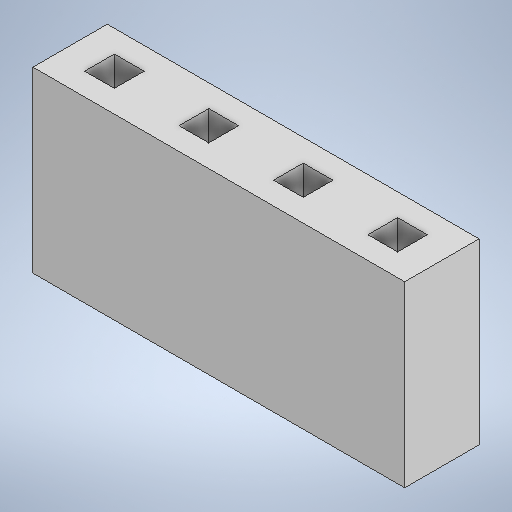
# Autodesk Inventor part: ikafly8_2.54
Saved by Autodesk Inventor 2025 (Build 290162000, 162)
## iProperties
Created: 2024-05-24
Part Number: ikafly8_2.54
Material: 一般
Document SubType Name: Modeling
Designer: Saigusa
Density: 1 g/cm^3
Appearance: 既定
Author: Saigusa
Autodesk Inventor part; units mm, degrees
ref_plane "YZ Plane" through (0, 0, 0) normal (1, 0, 0) x (0, 1, 0)
ref_plane "XZ Plane" through (0, 0, 0) normal (0, 1, 0) x (-1, 0, 0)
ref_plane "XY Plane" through (0, 0, 0) normal (0, 0, 1) x (1, 0, 0)
sketch "スケッチ1" plane through (0, 0, 0) normal (0, 1, 0) x (-1, 0, 0)
  line L0 (0, 0) -> (5.08, 0)
  line L1 (5.08, 0) -> (2.54, 0)
  line L2 (2.54, 0) -> (0, 0)
  line L3 (0, 0) -> (-2.54, 0)
  line L4 (-2.54, 0) -> (-5.08, 0)
  circle A0 centre (-2.54, 0) radius 0.4
  circle A1 centre (0, 0) radius 0.4
  circle A2 centre (2.54, 0) radius 0.4
  circle A3 centre (5.08, 0) radius 0.4
  line L5 (0, 0) -> (1.27, 0)
  line L6 (-3.73, -1) -> (6.27, -1)
  line L7 (6.27, -1) -> (6.27, 1)
  line L8 (6.27, 1) -> (-3.73, 1)
  line L9 (-3.73, 1) -> (-3.73, -1)
  line L10 (-3.73, -1) -> (6.27, 1) construction
  line L11 (6.27, -1) -> (-3.73, 1) construction
  line L12 (4.68, -0.4) -> (5.48, -0.4)
  line L13 (5.48, -0.4) -> (5.48, 0.4)
  line L14 (5.48, 0.4) -> (4.68, 0.4)
  line L15 (4.68, 0.4) -> (4.68, -0.4)
  line L16 (4.68, -0.4) -> (5.48, 0.4) construction
  line L17 (5.48, -0.4) -> (4.68, 0.4) construction
  line L18 (2.14, -0.4) -> (2.94, -0.4)
  line L19 (2.94, -0.4) -> (2.94, 0.4)
  line L20 (2.94, 0.4) -> (2.14, 0.4)
  line L21 (2.14, 0.4) -> (2.14, -0.4)
  line L22 (2.14, -0.4) -> (2.94, 0.4) construction
  line L23 (2.94, -0.4) -> (2.14, 0.4) construction
  line L24 (-0.4, -0.4) -> (0.4, -0.4)
  line L25 (0.4, -0.4) -> (0.4, 0.4)
  line L26 (0.4, 0.4) -> (-0.4, 0.4)
  line L27 (-0.4, 0.4) -> (-0.4, -0.4)
  line L28 (-0.4, -0.4) -> (0.4, 0.4) construction
  line L29 (0.4, -0.4) -> (-0.4, 0.4) construction
  line L30 (-2.94, -0.4) -> (-2.14, -0.4)
  line L31 (-2.14, -0.4) -> (-2.14, 0.4)
  line L32 (-2.14, 0.4) -> (-2.94, 0.4)
  line L33 (-2.94, 0.4) -> (-2.94, -0.4)
  line L34 (-2.94, -0.4) -> (-2.14, 0.4) construction
  line L35 (-2.14, -0.4) -> (-2.94, 0.4) construction
  dimension "d0" = 5.08
  dimension "d1" = 2.54
  dimension "d2" = 2.54
  dimension "d3" = 2.54
  dimension "d4" = 0.8
  dimension "d5" = 0.8
  dimension "d6" = 0.8
  dimension "d7" = 0.8
  dimension "d8" = 1.27
  dimension "d9" = 10
  dimension "d10" = 2
  constraints: 72 end point, 12 midpoint, 11 equal length, 6 horizontal, 5 perpendicular, 4 centre point, 4 coincident, 4 point on line
  measures "d0" distance of L0.start L0.end
  measures "d1" distance of L0.end L1.end
  measures "d2" distance of L0.start L3.end
  measures "d3" distance of L3.end L4.end
  measures "d4" diameter of A0
  measures "d5" diameter of A1
  measures "d6" diameter of A2
  measures "d7" diameter of A3
  measures "d8" distance of L5.start L5.end
  measures "d9" distance of L8.end L7.end
  measures "d10" distance of L7.end L6.end
extrude "押し出し1" add sketch "スケッチ1" along normal blind 4.8
